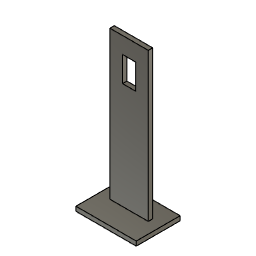
Holder motora kamere (Autodesk Fusion 360 design; units mm, degrees)
Autodesk Fusion 360 part; units mm, degrees
sketch "Sketch1" plane through (0, 0, 0) normal (0, 0, 1) x (1, 0, 0)
  line L0 (-17.5, -67.5) -> (-17.5, 67.5)
  line L1 (-17.5, 67.5) -> (17.5, 67.5)
  line L2 (17.5, 67.5) -> (17.5, -67.5)
  line L3 (-10, -67.5) -> (-10, -71.5)
  line L4 (-10, -71.5) -> (10, -71.5)
  line L5 (10, -71.5) -> (10, -67.5)
  line L6 (17.5, -67.5) -> (10, -67.5)
  line L7 (-10, -67.5) -> (-17.5, -67.5)
  line L8 (0, 52.5) -> (-6, 52.5)
  line L9 (-6, 52.5) -> (-6, 29.5)
  line L10 (-6, 29.5) -> (6, 29.5)
  line L11 (0, 52.5) -> (6, 52.5)
  line L12 (6, 52.5) -> (6, 29.5)
  dimension "d1" = 35
  dimension "d2" = 135
  dimension "d4" = 4
  dimension "d5" = 20
  dimension "d7" = 6
  dimension "d8" = 23
  dimension "d9" = 12
  dimension "d10" = 6
  constraint horizontal L6
  constraint perpendicular L0 L6
  constraint parallel L1 L6
  constraint parallel L0 L2
  constraint perpendicular L3 L6
  constraint perpendicular L3 L4
  constraint perpendicular L5 L6
  constraint collinear L6 L7
  constraint perpendicular L8 L9
  constraint perpendicular L9 L10
  measures "d1" distance of L0.end L1.end L5
  measures "d2" distance of L0.start L0.end L5
  measures "d4" distance of L3.start L3.end
  measures "d5" distance of L3.end L4.end
  measures "d7" distance of L8.start L8.end
  measures "d8" distance of L8.end L9.end
  measures "d9" distance of L9.end L10.end
  measures "d10" distance of L8.start L11.end
extrude "Extrude1" add sketch "Sketch1" along normal blind 4 makes body 1
sketch "Sketch2" plane through (0, 0, 0) normal (0, 0, 1) x (1, 0, 0)
  line L0 (167.5, -20) -> (112.5, -20)
  line L1 (112.5, -20) -> (112.5, 20)
  line L2 (112.5, 20) -> (167.5, 20)
  line L3 (167.5, 20) -> (167.5, -20)
  line L4 (167.5, -20) -> (112.5, 20) construction
  line L5 (112.5, -20) -> (167.5, 20) construction
  line L6 (140, 5) -> (130, 5)
  line L7 (130, 5) -> (130, 1)
  line L8 (130, 1) -> (150, 1)
  line L9 (150, 1) -> (150, 5)
  line L10 (150, 5) -> (140, 5)
  point P0 (140, 0)
  dimension "d13" = 55
  dimension "d14" = 40
  dimension "d16" = 10
  dimension "d17" = 4
  dimension "d18" = 20
  constraint horizontal L0
  constraint perpendicular L0 L1
  constraint parallel L0 L2
  constraint parallel L1 L3
  constraint coincident L4 P0
  constraint coincident L5 P0
  constraint perpendicular L6 L7
  constraint perpendicular L7 L8
  constraint perpendicular L8 L9
  measures "d4" distance of L8.end
  measures "d13" distance of L1.end L2.end
  measures "d14" distance of L0.end L1.end
  measures "d16" distance of L6.start L6.end
  measures "d17" distance of L6.end L7.end
  measures "d18" distance of L7.end L8.end
extrude "Extrude2" add sketch "Sketch2" along normal blind 4 separate body makes body 2
copy_body "Body->Comp1" bodies 2 removing the originals makes body 3 in component "Component"
move_body "Move1" bodies 1 to x (1, 0, 0) y (0, 0, 1) z (0, -1, 0) at (0, -65.5, 69.5)
move_body "Move1'" bodies 3 to x (1, 0, 0) y (0, 0, 1) z (0, -1, 0) at (0, 7, 1) in component "Component"
component "Component" placed x (1, 0, 0) y (0, 0, -1) z (0, 1, 0) at (-140, -71.5, 5)
